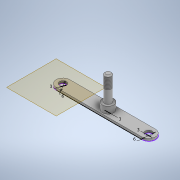
# Autodesk Inventor part: linkToActuator3
Saved by Autodesk Inventor 2021 (Build 250183000, 183)
## iProperties
Created: 2021-01-03
Part Number: linkToActuator3
Material: Generic
Document SubType Name: Modeling
Designer: awitc
Density: 1 g/cm^3
Appearance: Smooth - Medium Gray
Author: awitc
Autodesk Inventor part; units mm, degrees
ref_plane "YZ Plane" through (0, 0, 0) normal (1, 0, 0) x (0, 1, 0)
ref_plane "XZ Plane" through (0, 0, 0) normal (0, 1, 0) x (-1, 0, 0)
ref_plane "XY Plane" through (0, 0, 0) normal (0, 0, 1) x (1, 0, 0)
sketch "Sketch1" plane through (0, 0, 0) normal (0, 1, 0) x (-1, 0, 0)
  line L0 (0, -6) -> (0, 0)
  circle A0 centre (-20, -3) radius 1.5
  circle A1 centre (-38, -3) radius 1.5
  circle A2 centre (0, -3) radius 1.5
  circle A3 centre (0, -3) radius 3
  circle A4 centre (-38, -3) radius 3
  line L1 (-38, 0) -> (0, 0)
  line L2 (0, -6) -> (-38, -6)
  point P0 (0, -4.5)
  point P1 (0, -1.5)
  dimension "d11" = 3
  dimension "d26" = 3
  dimension "d27" = 3
  dimension "d28" = 6
  dimension "d29" = 6
  constraints: 6 end point, 5 centre point, 3 tangent, 2 coincident, 2 point on circle, 1 horizontal
  measures "d11" diameter of A0
  measures "d26" diameter of A1
  measures "d27" diameter of A2
  measures "d28" diameter of A3
  measures "d29" diameter of A4
extrude "Extrusion2" add sketch "Sketch1" along normal blind 15 contours A0
ref_plane "Work Plane1" through (0, 1, 0) normal (0, 1, 0) x (1, 0, 0)
sketch "Sketch2" plane through (0, 1, 0) normal (0, 1, 0) x (1, 0, 0)
  circle A0 centre (20, 3) radius 1.5 projected
  circle A1 centre (20, 3) radius 2.5
  circle A2 centre (20, 3) radius 1.5
  point P0 (0, 0)
  dimension "d14" = 5
  constraints: 2 centre point, 2 coincident
  measures "d14" diameter of A1
extrude "Extrusion3" add sketch "Sketch2" along normal blind 3
chamfer "Chamfer1" distance 0.5 angle 45 1 edges at (21.5, 15, -3)
extrude "Extrusion4" add sketch "Sketch1" along normal blind 1 contours A3 L0 A2 | L2 A4 L1 A3 | L0 A2 A3 | A4
thread "Thread2" size "M3x0.5" class "6g" standard "ANSI Metric M Profile" length 5
body "Solid1"
